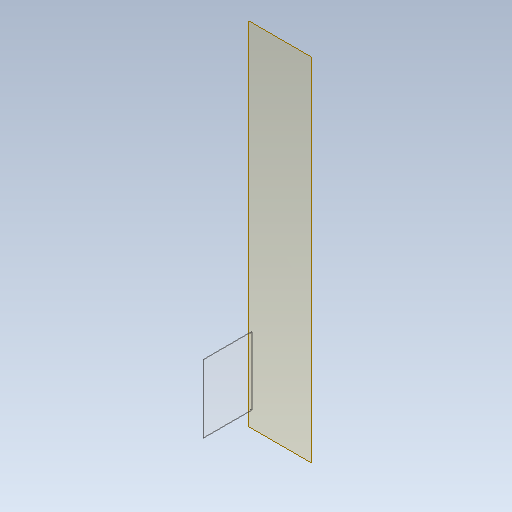
# Autodesk Inventor part: Barrera de protección
Saved by Autodesk Inventor 2021 (Build 250183000, 183)
## iProperties
Created: 2021-07-18
Part Number: Barrera de protección
Material: PMMA Plastic
Document SubType Name: Modeling
Designer: maaro
Density: 1.188 g/cm^3
Appearance: Polycarbonate - Clear
Author: maaro
Autodesk Inventor part; units mm, degrees
ref_plane "YZ Plane" through (0, 0, 0) normal (1, 0, 0) x (0, 1, 0)
ref_plane "XZ Plane" through (0, 0, 0) normal (0, 1, 0) x (-1, 0, 0)
ref_plane "XY Plane" through (0, 0, 0) normal (0, 0, 1) x (1, 0, 0)
ref_plane "Work Plane1" through (0, 0, 0) normal (0, 0, 1) x (1, 0, 0)
sketch "Sketch1" plane through (0, 0, 0) normal (0, 0, 1) x (1, 0, 0)
  line L0 (-590.856, -3290.856) -> (590.856, -3290.856) projected
  line L1 (-590.856, 3290.856) -> (-590.856, -3290.856) projected
  line L2 (-590.856, -3290.856) -> (-590.856, -1890.856)
  line L3 (-590.856, -1890.856) -> (-580.856, -1890.856)
  line L4 (-580.856, -1890.856) -> (-580.856, -3290.856)
  line L5 (-580.856, -3290.856) -> (-590.856, -3290.856)
  point P0 (0, 0)
  dimension "d0" = 1400
  dimension "d1" = 10
  constraints: 8 end point, 2 perpendicular, 2 point on line, 1 horizontal
  measures "d0" distance of L0.start L2.end
  measures "d1" distance of L2.end L3.end
extrude "Extrusion1" add sketch "Sketch1" along normal blind 1000
sketch "Sketch2" plane through (-590.856, -3290.856, 0) normal (-1, 0, 0) x (0, 0, 1)
  circle A0 centre (25, 1375) radius 3 projected
  circle A1 centre (25.1726, 25.0861) radius 3 projected
  point P0 (0, 3290.856)
extrude "Extrusion2" cut sketch "Sketch2" against normal through all
body "Solid1"
